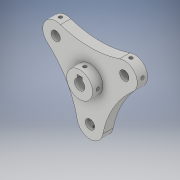
# Autodesk Inventor part: Stage1_carrier
Saved by Autodesk Inventor 2019 (Build 230136000, 136)
## iProperties
Created: 2019-12-31
Part Number: Stage1_carrier
Material: 一般
Document SubType Name: Modeling
Designer: user
Density: 1 g/cm^3
Appearance: 預設
Author: user
Autodesk Inventor part; units mm, degrees
note: some values were not read from the file. Chosen so that the rebuilt part matches the saved one: direction of "孔1"; direction of "孔2"; direction of "孔5".
sketch "草圖1" plane through (0, 0, 0) normal (0, 0, 1) x (1, 0, 0)
  arc A0 (0, -54.75) -> (10.672793, -53.699665) centre (0, 0) ccw
  circle A1 centre (-33.125472, 19.125) radius 12.5
  circle A2 centre (33.125472, 19.125) radius 12.5
  circle A3 centre (0, -38.25) radius 12.5
  line L0 (0, -92.899807) -> (0, 150.962186)
  arc A4 (-12.264267, -40.666144) -> (-41.350047, 9.711905) centre (-100.566991, -58.062379) ccw
  arc A5 (41.350047, 9.711905) -> (12.264267, -40.666144) centre (100.566991, -58.062379) ccw
  arc A6 (-29.08578, 30.954239) -> (29.08578, 30.954239) centre (0, 116.124758) ccw
  arc A7 (12.361843, -40.103334) -> (12.378027, -40.098341) centre (0, 0) ccw
  arc A8 (40.915196, 9.329485) -> (40.911427, 9.345997) centre (0, 0) ccw
  arc A9 (-40.911427, 9.345997) -> (-40.915196, 9.329485) centre (0, 0) ccw
  arc A10 (-12.378027, -40.098341) -> (-12.361843, -40.103334) centre (0, 0) ccw
  arc A11 (28.549585, 30.757337) -> (28.537169, 30.768856) centre (0, 0) ccw
  arc A12 (-28.537169, 30.768856) -> (-28.549585, 30.757337) centre (0, 0) ccw
  dimension "d0" = 109.5
  dimension "d6" = 25
  dimension "d10" = 38.25
  dimension "d11" = 90
  dimension "d12" = 90
  dimension "d13" = 33.12547
  dimension "d14" = 19.125
  dimension "d15" = 57.375
  dimension "d16" = 100.56699
  dimension "d17" = 9.4131
  constraints: 39 point on circle, 13 centre point, 6 tangent, 3 equal radius, 2 coincident, 2 point on line, 1 other
  measures "d0" diameter of A0
  measures "d6" diameter of A3
  measures "d10" distance of A3.centre point (0, 0)
  measures "d11" radius of A6
  measures "d12" radius of A5
  measures "d13" distance from line of L0 A1.centre
  measures "d14" vertical distance of point (0, 0) A1.centre
  measures "d15" vertical distance of A1.centre A3.centre
  measures "d16" horizontal distance of point (0, 0) A5.centre
  measures "d17" vertical distance of A2.start A2.centre
extrude "擠出1" add sketch "草圖1" along normal blind 10 contours A1 | A1 A12 A6 L0 A3 A10 A4 A9 | A6 A11 A2 A8 A5 A7 A3 L0 | L0 A3 | A3 L0 | A2
sketch "草圖2" plane through (0, 0, 10) normal (0, 0, 1) x (1, 0, 0)
  arc A0 (-28.549585, 30.757337) -> (-40.911427, 9.345997) centre (-33.125472, 19.125) ccw
  arc A1 (-28.549585, 30.757337) -> (-40.911427, 9.345997) centre (-33.125472, 19.125) ccw
  arc A2 (-40.911427, 9.345997) -> (-40.915196, 9.329485) centre (0, 0) ccw
  arc A3 (-12.378027, -40.098341) -> (-40.915196, 9.329485) centre (-100.566991, -58.062379) ccw
  arc A4 (-12.378027, -40.098341) -> (-12.361843, -40.103334) centre (0, 0) ccw
  arc A5 (-12.361843, -40.103334) -> (12.361843, -40.103334) centre (0, -38.25) ccw
  arc A6 (12.361843, -40.103334) -> (12.378027, -40.098341) centre (0, 0) ccw
  arc A7 (40.915196, 9.329485) -> (12.378027, -40.098341) centre (100.566991, -58.062379) ccw
  arc A8 (40.915196, 9.329485) -> (40.911427, 9.345997) centre (0, 0) ccw
  arc A9 (40.911427, 9.345997) -> (28.549585, 30.757337) centre (33.125472, 19.125) ccw
  arc A10 (28.549585, 30.757337) -> (28.537169, 30.768856) centre (0, 0) ccw
  arc A11 (-28.537169, 30.768856) -> (28.537169, 30.768856) centre (0, 116.124758) ccw
  arc A12 (-28.537169, 30.768856) -> (-28.549585, 30.757337) centre (0, 0) ccw
  arc A13 (40.911427, 9.345997) -> (28.549585, 30.757337) centre (33.125472, 19.125) ccw
  circle A14 centre (-33.125472, 19.125) radius 4.5
  circle A15 centre (33.125472, 19.125) radius 4.5
  circle A16 centre (0, -38.25) radius 4.5
  circle A17 centre (-33.125472, 19.125) radius 5
  circle A18 centre (33.125472, 19.125) radius 81.787496
  dimension "d20" = 9
  dimension "d46" = 10
  constraints: 5 centre point, 5 coincident, 2 equal radius
  measures "d20" diameter of A14
  measures "d46" diameter of A17
extrude "擠出2" cut sketch "草圖2" against normal up to surface (10 mm away) contours A14 | A15 | A16
sketch "草圖3" plane through (0, 0, 10) normal (0, 0, 1) x (1, 0, 0)
  circle A0 centre (0, 0) radius 5
  line L0 (-2.5, 4.330127) -> (-2.5, 7.330127)
  line L1 (-2.5, 7.330127) -> (2.5, 7.330127)
  line L2 (2.5, 7.330127) -> (2.5, 4.330127)
  line L3 (0, -67.225) -> (0, 48.1)
  circle A1 centre (0, 0) radius 10
  dimension "d23" = 10
  dimension "d26" = 5
  dimension "d27" = 3
  dimension "d28" = 20
  constraints: 6 end point, 2 centre point, 2 coincident, 2 perpendicular, 2 point on circle, 1 vertical, 1 other
  measures "d23" diameter of A0
  measures "d26" distance of L0.end L1.end
  measures "d27" distance of L1.end L2.end
  measures "d28" diameter of A1
extrude "擠出3" cut sketch "草圖3" against normal blind 10 contours A0 L3 | A0 L3 L1 L2 | A0 L3 | A0 L0 L1 L3
sketch "草圖4" plane through (0, 0, 10) normal (0, 0, 1) x (1, 0, 0)
  arc A0 (-2.5, 4.330127) -> (2.5, 4.330127) centre (0, 0) ccw
  arc A1 (-2.5, 4.330127) -> (2.5, 4.330127) centre (0, 0) ccw
  line L0 (-2.5, 4.330127) -> (-2.5, 7.330127)
  line L1 (-2.5, 7.330127) -> (2.5, 7.330127)
  line L2 (2.5, 7.330127) -> (2.5, 4.330127)
  circle A2 centre (33.125472, 19.125) radius 4.5
  circle A3 centre (0, -38.25) radius 4.5
  circle A4 centre (-33.125472, 19.125) radius 4.5
  arc A5 (-28.549585, 30.757337) -> (-40.911427, 9.345997) centre (-33.125472, 19.125) ccw
  arc A6 (-40.911427, 9.345997) -> (-40.915196, 9.329485) centre (0, 0) ccw
  arc A7 (-12.378027, -40.098341) -> (-40.915196, 9.329485) centre (-100.566991, -58.062379) ccw
  arc A8 (-12.378027, -40.098341) -> (-12.361843, -40.103334) centre (0, 0) ccw
  arc A9 (-12.361843, -40.103334) -> (12.361843, -40.103334) centre (0, -38.25) ccw
  arc A10 (12.361843, -40.103334) -> (12.378027, -40.098341) centre (0, 0) ccw
  arc A11 (40.915196, 9.329485) -> (12.378027, -40.098341) centre (100.566991, -58.062379) ccw
  arc A12 (40.915196, 9.329485) -> (40.911427, 9.345997) centre (0, 0) ccw
  arc A13 (40.911427, 9.345997) -> (28.549585, 30.757337) centre (33.125472, 19.125) ccw
  arc A14 (28.549585, 30.757337) -> (28.537169, 30.768856) centre (0, 0) ccw
  arc A15 (-28.537169, 30.768856) -> (28.537169, 30.768856) centre (0, 116.124758) ccw
  arc A16 (-28.537169, 30.768856) -> (-28.549585, 30.757337) centre (0, 0) ccw
  circle A17 centre (0, 0) radius 12.5
  dimension "d29" = 25
  constraints: 1 centre point, 1 coincident
  measures "d29" diameter of A17
extrude "擠出4" add sketch "草圖4" along normal blind 10 contours A17
ref_plane "工作平面1" through (0, 12.5, 10) normal (0, 1, 0) x (-1, 0, 0)
ref_plane "工作平面2" through (12.5, 0, 10) normal (1, 0, 0) x (0, 1, 0)
sketch "草圖5" plane through (0, 12.5, 10) normal (0, 1, 0) x (-1, 0, 0)
  point P0 (0, -10)
  point P1 (0, 5)
sketch "草圖6" plane through (12.5, 0, 10) normal (1, 0, 0) x (0, 1, 0)
  point P0 (0, -10)
  point P1 (0, 5)
hole "孔1" at (0, 12.5, 15) direction (0, -1, 0) diameter 3.242 depth 5.169873 thread size "M4x0.7" class "6H" standard "ISO Metric profile"
hole "孔2" at (12.5, 0, 15) direction (-1, 0, 0) diameter 3.242 end up to surface thread size "M4x0.7" class "6H" standard "ISO Metric profile"
ref_plane "工作平面4" through (45.625472, 19.125, 0) normal (1, 0, 0) x (0, 1, 0)
ref_plane "工作平面9" through (-45.625472, 19.125, 0) normal (1, 0, 0) x (0, 1, 0)
ref_plane "工作平面11" through (0, -50.75, 0) normal (0, 1, 0) x (-1, 0, 0)
ref_plane "工作平面10" through (-33.125472, 31.625, 0) normal (0, 1, 0) x (-1, 0, 0)
ref_plane "工作平面12" through (-12.5, -38.25, 0) normal (1, 0, 0) x (0, 1, 0)
sketch "草圖10" plane through (-45.625472, 19.125, 0) normal (1, 0, 0) x (0, 1, 0)
  line L0 (12.5, 0) -> (12.5, 10) projected
  point P0 (-19.125, 0)
  point P1 (1.580308, 4.885702)
sketch "草圖11" plane through (-33.125472, 31.625, 0) normal (0, 1, 0) x (-1, 0, 0)
  point P0 (-33.125472, 0)
  point P1 (-74.017675, 5)
  point P2 (0.911678, 4.536513)
sketch "草圖14" plane through (0, -50.75, 0) normal (0, 1, 0) x (-1, 0, 0)
  line L0 (-12.5, 10) -> (12.5, 10) projected
  point P0 (0, 0)
  point P1 (-13.541322, -36.353523)
  point P2 (0, 5)
hole "孔3" at (0, -50.75, 5) direction (0, 1, 0) diameter 3.242 end up to surface thread size "M4x0.7" class "6H" standard "ISO Metric profile"
hole "孔4" at (-45.625472, 20.705308, 4.885702) direction (1, 0, 0) diameter 3.242 end up to surface thread size "M4x0.7" class "6H" standard "ISO Metric profile"
mirror "鏡射1" about plane through (0, 0, 0) normal (1, 0, 0) of "孔4"
hole "孔5" at (-34.03715, 31.625, 4.536513) direction (0, -1, 0) diameter 3.242 end up to surface thread size "M4x0.7" class "6H" standard "ISO Metric profile"
mirror "鏡射2" about plane through (0, 0, 0) normal (1, 0, 0) of "孔5"
ref_plane "工作平面14" through (-190.566991, -58.062379, 0) normal (1, 0, 0) x (0, 1, 0)
ref_plane "工作平面15" through (-18.75, -38.25, 0) normal (1, 0, 0) x (0, 1, 0)
sketch "草圖16" plane through (-18.75, -38.25, 0) normal (1, 0, 0) x (0, 1, 0)
  point P0 (38.25, 0)
  point P1 (-0.012598, 5.096671)
hole "孔7" at (-18.75, -38.262598, 5.096671) direction (1, 0, 0) diameter 3.242 depth 14.87272 tip angle 118 thread size "M4x0.7" class "6H" standard "ISO Metric profile"
ref_plane "工作平面13" through (0, 0, 0) normal (1, 0, 0) x (0, 1, 0)
